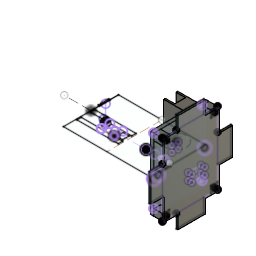
Slider Gear and Screw Box (Autodesk Fusion 360 design; units mm, degrees)
description: Spur Gear; Module: 3.0; Num Teeth: 12; Pressure Angle: 20.0; Backlash: 0.00 mm
part number: 2026-03-27-17-39-36-868
Autodesk Fusion 360 part; units mm, degrees
(part 1 of 2)
sketch "Base Circle" plane through (0, 0, 0) normal (0, 0, 1) x (1, 0, 0)
  circle A0 centre (0, 0) radius 14.529
  circle A1 centre (0, 0) radius 1.75
  dimension "d22" = 3.5
  measures "d22" diameter of A1
extrude "Extrude1" add sketch "Base Circle" along normal blind 8 makes body 1
sketch "Gear Tooth" plane through (0, 0, 0) normal (0, 0, 1) x (1, 0, 0)
  spline S0 degree 5 poles (16.735, -2.4575) (16.7471, -2.4592) (16.7712, -2.4624) (16.8075, -2.466) (16.8561, -2.4685) (16.9171, -2.4687) (16.9782, -2.4667) (17.0395, -2.4633) (17.1009, -2.4593) (17.1623, -2.4548) (17.2237, -2.4497) (17.2852, -2.4439) (17.3467, -2.4372) (17.4083, -2.4294) (17.4699, -2.4206) (17.5316, -2.4107) (17.5933, -2.4) (17.6549, -2.3886) (17.7166, -2.3766) (17.7783, -2.364) (17.84, -2.3508) (17.9017, -2.337) (17.9634, -2.3225) (18.025, -2.3073) (18.0867, -2.2914) (18.1483, -2.2749) (18.2099, -2.2578) (18.2715, -2.2401) (18.3331, -2.2219) (18.3946, -2.2031) (18.4561, -2.1837) (18.5175, -2.1638) (18.579, -2.1433) (18.6403, -2.1223) (18.7017, -2.1007) (18.763, -2.0786) (18.8242, -2.056) (18.8854, -2.0329) (18.9465, -2.0092) (19.0076, -1.9851) (19.0686, -1.9605) (19.1296, -1.9353) (19.1905, -1.9097) (19.2514, -1.8836) (19.3121, -1.857) (19.3728, -1.8299) (19.4335, -1.8024) (19.494, -1.7743) (19.5545, -1.7459) (19.615, -1.7169) (19.6753, -1.6875) (19.7355, -1.6577) (19.7957, -1.6274) (19.8558, -1.5966) (19.9158, -1.5654) (19.9757, -1.5338) (20.0356, -1.5017) (20.0953, -1.4692) (20.155, -1.4362) (20.2145, -1.4029) (20.274, -1.3691) (20.3333, -1.3348) (20.3926, -1.3002) (20.4518, -1.2651) (20.5108, -1.2296) (20.5698, -1.1937) (20.6286, -1.1574) (20.6874, -1.1207) (20.746, -1.0836) (20.8045, -1.0461) (20.8629, -1.0082) (20.9095, -0.9775) (20.9445, -0.9544) (20.9677, -0.9388) (20.9794, -0.931) knots 0 0 0 0 0 0 0.01428571 0.02857143 0.04285714 0.05714286 0.07142857 0.08571429 0.1 0.11428571 0.12857143 0.14285714 0.15714286 0.17142857 0.18571429 0.2 0.21428571 0.22857143 0.24285714 0.25714286 0.27142857 0.28571429 0.3 0.31428571 0.32857143 0.34285714 0.35714286 0.37142857 0.38571429 0.4 0.41428571 0.42857143 0.44285714 0.45714286 0.47142857 0.48571429 0.5 0.51428571 0.52857143 0.54285714 0.55714286 0.57142857 0.58571429 0.6 0.61428571 0.62857143 0.64285714 0.65714286 0.67142857 0.68571429 0.7 0.71428571 0.72857143 0.74285714 0.75714286 0.77142857 0.78571429 0.8 0.81428571 0.82857143 0.84285714 0.85714286 0.87142857 0.88571429 0.9 0.91428571 0.92857143 0.94285714 0.95714286 0.97142857 0.98571429 1 1 1 1 1 1
  spline S1 degree 5 poles (16.735, 2.4575) (16.7471, 2.4592) (16.7712, 2.4624) (16.8075, 2.466) (16.8561, 2.4685) (16.9171, 2.4687) (16.9782, 2.4667) (17.0395, 2.4633) (17.1009, 2.4593) (17.1623, 2.4548) (17.2237, 2.4497) (17.2852, 2.4439) (17.3467, 2.4372) (17.4083, 2.4294) (17.4699, 2.4206) (17.5316, 2.4107) (17.5933, 2.4) (17.6549, 2.3886) (17.7166, 2.3766) (17.7783, 2.364) (17.84, 2.3508) (17.9017, 2.337) (17.9634, 2.3225) (18.025, 2.3073) (18.0867, 2.2914) (18.1483, 2.2749) (18.2099, 2.2578) (18.2715, 2.2401) (18.3331, 2.2219) (18.3946, 2.2031) (18.4561, 2.1837) (18.5175, 2.1638) (18.579, 2.1433) (18.6403, 2.1223) (18.7017, 2.1007) (18.763, 2.0786) (18.8242, 2.056) (18.8854, 2.0329) (18.9465, 2.0092) (19.0076, 1.9851) (19.0686, 1.9605) (19.1296, 1.9353) (19.1905, 1.9097) (19.2514, 1.8836) (19.3121, 1.857) (19.3728, 1.8299) (19.4335, 1.8024) (19.494, 1.7743) (19.5545, 1.7459) (19.615, 1.7169) (19.6753, 1.6875) (19.7355, 1.6577) (19.7957, 1.6274) (19.8558, 1.5966) (19.9158, 1.5654) (19.9757, 1.5338) (20.0356, 1.5017) (20.0953, 1.4692) (20.155, 1.4362) (20.2145, 1.4029) (20.274, 1.3691) (20.3333, 1.3348) (20.3926, 1.3002) (20.4518, 1.2651) (20.5108, 1.2296) (20.5698, 1.1937) (20.6286, 1.1574) (20.6874, 1.1207) (20.746, 1.0836) (20.8045, 1.0461) (20.8629, 1.0082) (20.9095, 0.9775) (20.9445, 0.9544) (20.9677, 0.9388) (20.9794, 0.931) knots 0 0 0 0 0 0 0.01428571 0.02857143 0.04285714 0.05714286 0.07142857 0.08571429 0.1 0.11428571 0.12857143 0.14285714 0.15714286 0.17142857 0.18571429 0.2 0.21428571 0.22857143 0.24285714 0.25714286 0.27142857 0.28571429 0.3 0.31428571 0.32857143 0.34285714 0.35714286 0.37142857 0.38571429 0.4 0.41428571 0.42857143 0.44285714 0.45714286 0.47142857 0.48571429 0.5 0.51428571 0.52857143 0.54285714 0.55714286 0.57142857 0.58571429 0.6 0.61428571 0.62857143 0.64285714 0.65714286 0.67142857 0.68571429 0.7 0.71428571 0.72857143 0.74285714 0.75714286 0.77142857 0.78571429 0.8 0.81428571 0.82857143 0.84285714 0.85714286 0.87142857 0.88571429 0.9 0.91428571 0.92857143 0.94285714 0.95714286 0.97142857 0.98571429 1 1 1 1 1 1
  arc A0 (20.9794, -0.931) -> (20.9794, 0.931) centre (0, 0) ccw
  line L0 (14.3649, -2.1094) -> (16.735, -2.4575)
  line L1 (14.3649, 2.1094) -> (16.735, 2.4575)
  line L2 (14.3649, -2.1094) -> (14.3649, 2.1094)
  point P0 (17.029, -2.4638)
  point P1 (17.3273, -2.4392)
  point P2 (17.6282, -2.3935)
  point P3 (17.931, -2.33)
  point P4 (18.2352, -2.2505)
  point P5 (18.5405, -2.1561)
  point P6 (18.8463, -2.0476)
  point P7 (19.1525, -1.9256)
  point P8 (19.4587, -1.7906)
  point P9 (19.7645, -1.643)
  point P10 (20.0698, -1.483)
  point P11 (20.3742, -1.3109)
  point P12 (20.6775, -1.1268)
  point P13 (17.029, 2.4638)
  point P14 (17.3273, 2.4392)
  point P15 (17.6282, 2.3935)
  point P16 (17.931, 2.33)
  point P17 (18.2352, 2.2505)
  point P18 (18.5405, 2.1561)
  point P19 (18.8463, 2.0476)
  point P20 (19.1525, 1.9256)
  point P21 (19.4587, 1.7906)
  point P22 (19.7645, 1.643)
  point P23 (20.0698, 1.483)
  point P24 (20.3742, 1.3109)
  point P25 (20.6775, 1.1268)
extrude "Extrude2" add sketch "Gear Tooth" along normal blind 8 bodies 1
fillet "Fillet1" radius 1 2 edges at (14.3748, -2.1109, 4) (14.3748, 2.1109, 4) on bodies 1
pattern_circular "C-Pattern1" count 12 over 360 about axis through (0, 0, 0) along (0, 0, 1) of "Extrude2", "Fillet1"
sketch "Diametrial Pitch Circle" plane through (0, 0, 0) normal (0, 0, 1) x (1, 0, 0)
  circle A0 centre (0, 0) radius 18 construction
sketch "Connecting Rod" plane through (0, 0, 8) normal (0, 0, 1) x (-1, 0, 0)
  arc A0 (-13.8215, 4.4786) -> (-14.2091, 3.0322) centre (0, 0) ccw
  arc A1 (-15.3323, 2.2515) -> (-14.2091, 3.0322) centre (-15.1871, 3.2409) ccw
  line L0 (-15.3323, 2.2515) -> (-16.735, 2.4575)
  spline S0 degree 5 poles (-16.735, 2.4575) (-16.7471, 2.4592) (-16.7712, 2.4624) (-16.8075, 2.466) (-16.8561, 2.4685) (-16.9171, 2.4687) (-16.9782, 2.4667) (-17.0395, 2.4633) (-17.1009, 2.4593) (-17.1623, 2.4548) (-17.2237, 2.4497) (-17.2852, 2.4439) (-17.3467, 2.4372) (-17.4083, 2.4294) (-17.4699, 2.4206) (-17.5316, 2.4107) (-17.5933, 2.4) (-17.6549, 2.3886) (-17.7166, 2.3766) (-17.7783, 2.364) (-17.84, 2.3508) (-17.9017, 2.337) (-17.9634, 2.3225) (-18.025, 2.3073) (-18.0867, 2.2914) (-18.1483, 2.2749) (-18.2099, 2.2578) (-18.2715, 2.2401) (-18.3331, 2.2219) (-18.3946, 2.2031) (-18.4561, 2.1837) (-18.5175, 2.1638) (-18.579, 2.1433) (-18.6403, 2.1223) (-18.7017, 2.1007) (-18.763, 2.0786) (-18.8242, 2.056) (-18.8854, 2.0329) (-18.9465, 2.0092) (-19.0076, 1.9851) (-19.0686, 1.9605) (-19.1296, 1.9353) (-19.1905, 1.9097) (-19.2514, 1.8836) (-19.3121, 1.857) (-19.3728, 1.8299) (-19.4335, 1.8024) (-19.494, 1.7743) (-19.5545, 1.7459) (-19.615, 1.7169) (-19.6753, 1.6875) (-19.7355, 1.6577) (-19.7957, 1.6274) (-19.8558, 1.5966) (-19.9158, 1.5654) (-19.9757, 1.5338) (-20.0356, 1.5017) (-20.0953, 1.4692) (-20.155, 1.4362) (-20.2145, 1.4029) (-20.274, 1.3691) (-20.3333, 1.3348) (-20.3926, 1.3002) (-20.4518, 1.2651) (-20.5108, 1.2296) (-20.5698, 1.1937) (-20.6286, 1.1574) (-20.6874, 1.1207) (-20.746, 1.0836) (-20.8045, 1.0461) (-20.8629, 1.0082) (-20.9095, 0.9775) (-20.9445, 0.9544) (-20.9677, 0.9388) (-20.9794, 0.931) knots 0 0 0 0 0 0 0.01428571 0.02857143 0.04285714 0.05714286 0.07142857 0.08571429 0.1 0.11428571 0.12857143 0.14285714 0.15714286 0.17142857 0.18571429 0.2 0.21428571 0.22857143 0.24285714 0.25714286 0.27142857 0.28571429 0.3 0.31428571 0.32857143 0.34285714 0.35714286 0.37142857 0.38571429 0.4 0.41428571 0.42857143 0.44285714 0.45714286 0.47142857 0.48571429 0.5 0.51428571 0.52857143 0.54285714 0.55714286 0.57142857 0.58571429 0.6 0.61428571 0.62857143 0.64285714 0.65714286 0.67142857 0.68571429 0.7 0.71428571 0.72857143 0.74285714 0.75714286 0.77142857 0.78571429 0.8 0.81428571 0.82857143 0.84285714 0.85714286 0.87142857 0.88571429 0.9 0.91428571 0.92857143 0.94285714 0.95714286 0.97142857 0.98571429 1 1 1 1 1 1
  arc A2 (-20.9794, 0.931) -> (-20.9794, -0.931) centre (0, 0) ccw
  spline S1 degree 5 poles (-20.9794, -0.931) (-20.9677, -0.9388) (-20.9445, -0.9544) (-20.9095, -0.9775) (-20.8629, -1.0082) (-20.8045, -1.0461) (-20.746, -1.0836) (-20.6874, -1.1207) (-20.6286, -1.1574) (-20.5698, -1.1937) (-20.5108, -1.2296) (-20.4518, -1.2651) (-20.3926, -1.3002) (-20.3333, -1.3348) (-20.274, -1.3691) (-20.2145, -1.4029) (-20.155, -1.4362) (-20.0953, -1.4692) (-20.0356, -1.5017) (-19.9757, -1.5338) (-19.9158, -1.5654) (-19.8558, -1.5966) (-19.7957, -1.6274) (-19.7355, -1.6577) (-19.6753, -1.6875) (-19.615, -1.7169) (-19.5545, -1.7459) (-19.494, -1.7743) (-19.4335, -1.8024) (-19.3728, -1.8299) (-19.3121, -1.857) (-19.2514, -1.8836) (-19.1905, -1.9097) (-19.1296, -1.9353) (-19.0686, -1.9605) (-19.0076, -1.9851) (-18.9465, -2.0092) (-18.8854, -2.0329) (-18.8242, -2.056) (-18.763, -2.0786) (-18.7017, -2.1007) (-18.6403, -2.1223) (-18.579, -2.1433) (-18.5175, -2.1638) (-18.4561, -2.1837) (-18.3946, -2.2031) (-18.3331, -2.2219) (-18.2715, -2.2401) (-18.2099, -2.2578) (-18.1483, -2.2749) (-18.0867, -2.2914) (-18.025, -2.3073) (-17.9634, -2.3225) (-17.9017, -2.337) (-17.84, -2.3508) (-17.7783, -2.364) (-17.7166, -2.3766) (-17.6549, -2.3886) (-17.5933, -2.4) (-17.5316, -2.4107) (-17.4699, -2.4206) (-17.4083, -2.4294) (-17.3467, -2.4372) (-17.2852, -2.4439) (-17.2237, -2.4497) (-17.1623, -2.4548) (-17.1009, -2.4593) (-17.0395, -2.4633) (-16.9782, -2.4667) (-16.9171, -2.4687) (-16.8561, -2.4685) (-16.8075, -2.466) (-16.7712, -2.4624) (-16.7471, -2.4592) (-16.735, -2.4575) knots -1 -1 -1 -1 -1 -1 -0.98571429 -0.97142857 -0.95714286 -0.94285714 -0.92857143 -0.91428571 -0.9 -0.88571429 -0.87142857 -0.85714286 -0.84285714 -0.82857143 -0.81428571 -0.8 -0.78571429 -0.77142857 -0.75714286 -0.74285714 -0.72857143 -0.71428571 -0.7 -0.68571429 -0.67142857 -0.65714286 -0.64285714 -0.62857143 -0.61428571 -0.6 -0.58571429 -0.57142857 -0.55714286 -0.54285714 -0.52857143 -0.51428571 -0.5 -0.48571429 -0.47142857 -0.45714286 -0.44285714 -0.42857143 -0.41428571 -0.4 -0.38571429 -0.37142857 -0.35714286 -0.34285714 -0.32857143 -0.31428571 -0.3 -0.28571429 -0.27142857 -0.25714286 -0.24285714 -0.22857143 -0.21428571 -0.2 -0.18571429 -0.17142857 -0.15714286 -0.14285714 -0.12857143 -0.11428571 -0.1 -0.08571429 -0.07142857 -0.05714286 -0.04285714 -0.02857143 -0.01428571 0 0 0 0 0 0
  line L1 (-16.735, -2.4575) -> (-15.3323, -2.2515)
  arc A3 (-14.2091, -3.0322) -> (-15.3323, -2.2515) centre (-15.1871, -3.2409) ccw
  arc A4 (-14.4039, -5.7163) -> (-13.8215, -4.4786) centre (-14.7728, -4.7868) ccw
  line L2 (-14.4039, -5.7163) -> (-15.7217, -6.2393)
  spline S2 degree 5 poles (-15.7217, -6.2393) (-15.733, -6.2438) (-15.7555, -6.2531) (-15.7887, -6.2682) (-15.8321, -6.2903) (-15.885, -6.3206) (-15.9369, -6.3529) (-15.9883, -6.3864) (-16.0394, -6.4206) (-16.0903, -6.4553) (-16.141, -6.4904) (-16.1914, -6.5261) (-16.2413, -6.5627) (-16.2907, -6.6002) (-16.3397, -6.6387) (-16.3882, -6.678) (-16.4362, -6.7181) (-16.4839, -6.7588) (-16.5314, -6.8001) (-16.5785, -6.8418) (-16.6253, -6.8841) (-16.6718, -6.927) (-16.718, -6.9703) (-16.7638, -7.0143) (-16.8092, -7.0589) (-16.8544, -7.104) (-16.8992, -7.1496) (-16.9436, -7.1957) (-16.9878, -7.2423) (-17.0317, -7.2894) (-17.0753, -7.3369) (-17.1185, -7.3849) (-17.1615, -7.4333) (-17.2042, -7.4822) (-17.2465, -7.5315) (-17.2885, -7.5813) (-17.3303, -7.6315) (-17.3717, -7.6822) (-17.4128, -7.7332) (-17.4536, -7.7847) (-17.4942, -7.8365) (-17.5344, -7.8888) (-17.5743, -7.9414) (-17.614, -7.9944) (-17.6533, -8.0479) (-17.6923, -8.1017) (-17.7311, -8.1559) (-17.7695, -8.2104) (-17.8077, -8.2653) (-17.8455, -8.3206) (-17.8831, -8.3762) (-17.9203, -8.4322) (-17.9573, -8.4885) (-17.9939, -8.5452) (-18.0303, -8.6022) (-18.0664, -8.6596) (-18.1022, -8.7173) (-18.1376, -8.7753) (-18.1728, -8.8337) (-18.2077, -8.8924) (-18.2423, -8.9514) (-18.2766, -9.0107) (-18.3106, -9.0703) (-18.3443, -9.1303) (-18.3777, -9.1905) (-18.4108, -9.2511) (-18.4436, -9.3119) (-18.4761, -9.3731) (-18.5084, -9.4345) (-18.5403, -9.4963) (-18.5719, -9.5583) (-18.597, -9.6082) (-18.6156, -9.6457) (-18.628, -9.6708) (-18.6342, -9.6834) knots 0 0 0 0 0 0 0.01428571 0.02857143 0.04285714 0.05714286 0.07142857 0.08571429 0.1 0.11428571 0.12857143 0.14285714 0.15714286 0.17142857 0.18571429 0.2 0.21428571 0.22857143 0.24285714 0.25714286 0.27142857 0.28571429 0.3 0.31428571 0.32857143 0.34285714 0.35714286 0.37142857 0.38571429 0.4 0.41428571 0.42857143 0.44285714 0.45714286 0.47142857 0.48571429 0.5 0.51428571 0.52857143 0.54285714 0.55714286 0.57142857 0.58571429 0.6 0.61428571 0.62857143 0.64285714 0.65714286 0.67142857 0.68571429 0.7 0.71428571 0.72857143 0.74285714 0.75714286 0.77142857 0.78571429 0.8 0.81428571 0.82857143 0.84285714 0.85714286 0.87142857 0.88571429 0.9 0.91428571 0.92857143 0.94285714 0.95714286 0.97142857 0.98571429 1 1 1 1 1 1
  arc A5 (-18.6342, -9.6834) -> (-17.7031, -11.296) centre (0, 0) ccw
  spline S3 degree 5 poles (-17.7031, -11.296) (-17.6892, -11.2969) (-17.6613, -11.2987) (-17.6194, -11.3013) (-17.5637, -11.3046) (-17.4942, -11.3082) (-17.4247, -11.3114) (-17.3554, -11.3143) (-17.2862, -11.3167) (-17.2171, -11.3187) (-17.1481, -11.3203) (-17.0792, -11.3215) (-17.0104, -11.3223) (-16.9418, -11.3227) (-16.8733, -11.3226) (-16.8049, -11.3222) (-16.7366, -11.3213) (-16.6685, -11.32) (-16.6005, -11.3183) (-16.5326, -11.3161) (-16.4649, -11.3136) (-16.3973, -11.3106) (-16.3299, -11.3072) (-16.2627, -11.3033) (-16.1955, -11.2991) (-16.1286, -11.2944) (-16.0618, -11.2892) (-15.9952, -11.2836) (-15.9287, -11.2776) (-15.8624, -11.2712) (-15.7963, -11.2643) (-15.7304, -11.2569) (-15.6646, -11.2491) (-15.5991, -11.2408) (-15.5337, -11.2321) (-15.4685, -11.223) (-15.4036, -11.2133) (-15.3388, -11.2032) (-15.2742, -11.1927) (-15.2099, -11.1816) (-15.1458, -11.1701) (-15.0819, -11.1581) (-15.0182, -11.1456) (-14.9548, -11.1327) (-14.8916, -11.1192) (-14.8286, -11.1052) (-14.766, -11.0907) (-14.7035, -11.0758) (-14.6413, -11.0603) (-14.5794, -11.0443) (-14.5178, -11.0278) (-14.4565, -11.0107) (-14.3955, -10.993) (-14.3348, -10.9747) (-14.2745, -10.9559) (-14.2145, -10.9365) (-14.1547, -10.9165) (-14.0953, -10.8961) (-14.0362, -10.8751) (-13.9774, -10.8535) (-13.9191, -10.8312) (-13.8613, -10.8081) (-13.8041, -10.7841) (-13.7475, -10.7591) (-13.6913, -10.7334) (-13.6356, -10.707) (-13.5801, -10.6803) (-13.525, -10.6531) (-13.4703, -10.6253) (-13.4163, -10.5965) (-13.3636, -10.5658) (-13.3228, -10.5393) (-13.2931, -10.5181) (-13.2738, -10.5033) (-13.2642, -10.4957) knots -1 -1 -1 -1 -1 -1 -0.98571429 -0.97142857 -0.95714286 -0.94285714 -0.92857143 -0.91428571 -0.9 -0.88571429 -0.87142857 -0.85714286 -0.84285714 -0.82857143 -0.81428571 -0.8 -0.78571429 -0.77142857 -0.75714286 -0.74285714 -0.72857143 -0.71428571 -0.7 -0.68571429 -0.67142857 -0.65714286 -0.64285714 -0.62857143 -0.61428571 -0.6 -0.58571429 -0.57142857 -0.55714286 -0.54285714 -0.52857143 -0.51428571 -0.5 -0.48571429 -0.47142857 -0.45714286 -0.44285714 -0.42857143 -0.41428571 -0.4 -0.38571429 -0.37142857 -0.35714286 -0.34285714 -0.32857143 -0.31428571 -0.3 -0.28571429 -0.27142857 -0.25714286 -0.24285714 -0.22857143 -0.21428571 -0.2 -0.18571429 -0.17142857 -0.15714286 -0.14285714 -0.12857143 -0.11428571 -0.1 -0.08571429 -0.07142857 -0.05714286 -0.04285714 -0.02857143 -0.01428571 0 0 0 0 0 0
  line L3 (-13.2642, -10.4957) -> (-12.1524, -9.616)
  arc A6 (-10.7893, -9.7305) -> (-12.1524, -9.616) centre (-11.5319, -10.4002) ccw
  arc A7 (-9.616, -12.1524) -> (-9.7305, -10.7893) centre (-10.4002, -11.5319) ccw
  line L4 (-9.616, -12.1524) -> (-10.4957, -13.2642)
  spline S4 degree 5 poles (-10.4957, -13.2642) (-10.5033, -13.2738) (-10.5181, -13.2931) (-10.5393, -13.3228) (-10.5658, -13.3636) (-10.5965, -13.4163) (-10.6253, -13.4703) (-10.6531, -13.525) (-10.6803, -13.5801) (-10.707, -13.6356) (-10.7334, -13.6913) (-10.7591, -13.7475) (-10.7841, -13.8041) (-10.8081, -13.8613) (-10.8312, -13.9191) (-10.8535, -13.9774) (-10.8751, -14.0362) (-10.8961, -14.0953) (-10.9165, -14.1547) (-10.9365, -14.2145) (-10.9559, -14.2745) (-10.9747, -14.3348) (-10.993, -14.3955) (-11.0107, -14.4565) (-11.0278, -14.5178) (-11.0443, -14.5794) (-11.0603, -14.6413) (-11.0758, -14.7035) (-11.0907, -14.766) (-11.1052, -14.8286) (-11.1192, -14.8916) (-11.1327, -14.9548) (-11.1456, -15.0182) (-11.1581, -15.0819) (-11.1701, -15.1458) (-11.1816, -15.2099) (-11.1927, -15.2742) (-11.2032, -15.3388) (-11.2133, -15.4036) (-11.223, -15.4685) (-11.2321, -15.5337) (-11.2408, -15.5991) (-11.2491, -15.6646) (-11.2569, -15.7304) (-11.2643, -15.7963) (-11.2712, -15.8624) (-11.2776, -15.9287) (-11.2836, -15.9952) (-11.2892, -16.0618) (-11.2944, -16.1286) (-11.2991, -16.1955) (-11.3033, -16.2627) (-11.3072, -16.3299) (-11.3106, -16.3973) (-11.3136, -16.4649) (-11.3161, -16.5326) (-11.3183, -16.6005) (-11.32, -16.6685) (-11.3213, -16.7366) (-11.3222, -16.8049) (-11.3226, -16.8733) (-11.3227, -16.9418) (-11.3223, -17.0104) (-11.3215, -17.0792) (-11.3203, -17.1481) (-11.3187, -17.2171) (-11.3167, -17.2862) (-11.3143, -17.3554) (-11.3114, -17.4247) (-11.3082, -17.4942) (-11.3046, -17.5637) (-11.3013, -17.6194) (-11.2987, -17.6613) (-11.2969, -17.6892) (-11.296, -17.7031) knots 0 0 0 0 0 0 0.01428571 0.02857143 0.04285714 0.05714286 0.07142857 0.08571429 0.1 0.11428571 0.12857143 0.14285714 0.15714286 0.17142857 0.18571429 0.2 0.21428571 0.22857143 0.24285714 0.25714286 0.27142857 0.28571429 0.3 0.31428571 0.32857143 0.34285714 0.35714286 0.37142857 0.38571429 0.4 0.41428571 0.42857143 0.44285714 0.45714286 0.47142857 0.48571429 0.5 0.51428571 0.52857143 0.54285714 0.55714286 0.57142857 0.58571429 0.6 0.61428571 0.62857143 0.64285714 0.65714286 0.67142857 0.68571429 0.7 0.71428571 0.72857143 0.74285714 0.75714286 0.77142857 0.78571429 0.8 0.81428571 0.82857143 0.84285714 0.85714286 0.87142857 0.88571429 0.9 0.91428571 0.92857143 0.94285714 0.95714286 0.97142857 0.98571429 1 1 1 1 1 1
  arc A8 (-11.296, -17.7031) -> (-9.6834, -18.6342) centre (0, 0) ccw
  spline S5 degree 5 poles (-9.6834, -18.6342) (-9.6708, -18.628) (-9.6457, -18.6156) (-9.6082, -18.597) (-9.5583, -18.5719) (-9.4963, -18.5403) (-9.4345, -18.5084) (-9.3731, -18.4761) (-9.3119, -18.4436) (-9.2511, -18.4108) (-9.1905, -18.3777) (-9.1303, -18.3443) (-9.0703, -18.3106) (-9.0107, -18.2766) (-8.9514, -18.2423) (-8.8924, -18.2077) (-8.8337, -18.1728) (-8.7753, -18.1376) (-8.7173, -18.1022) (-8.6596, -18.0664) (-8.6022, -18.0303) (-8.5452, -17.9939) (-8.4885, -17.9573) (-8.4322, -17.9203) (-8.3762, -17.8831) (-8.3206, -17.8455) (-8.2653, -17.8077) (-8.2104, -17.7695) (-8.1559, -17.7311) (-8.1017, -17.6923) (-8.0479, -17.6533) (-7.9944, -17.614) (-7.9414, -17.5743) (-7.8888, -17.5344) (-7.8365, -17.4942) (-7.7847, -17.4536) (-7.7332, -17.4128) (-7.6822, -17.3717) (-7.6315, -17.3303) (-7.5813, -17.2885) (-7.5315, -17.2465) (-7.4822, -17.2042) (-7.4333, -17.1615) (-7.3849, -17.1185) (-7.3369, -17.0753) (-7.2894, -17.0317) (-7.2423, -16.9878) (-7.1957, -16.9436) (-7.1496, -16.8992) (-7.104, -16.8544) (-7.0589, -16.8092) (-7.0143, -16.7638) (-6.9703, -16.718) (-6.927, -16.6718) (-6.8841, -16.6253) (-6.8418, -16.5785) (-6.8001, -16.5314) (-6.7588, -16.4839) (-6.7181, -16.4362) (-6.678, -16.3882) (-6.6387, -16.3397) (-6.6002, -16.2907) (-6.5627, -16.2413) (-6.5261, -16.1914) (-6.4904, -16.141) (-6.4553, -16.0903) (-6.4206, -16.0394) (-6.3864, -15.9883) (-6.3529, -15.9369) (-6.3206, -15.885) (-6.2903, -15.8321) (-6.2682, -15.7887) (-6.2531, -15.7555) (-6.2438, -15.733) (-6.2393, -15.7217) knots -1 -1 -1 -1 -1 -1 -0.98571429 -0.97142857 -0.95714286 -0.94285714 -0.92857143 -0.91428571 -0.9 -0.88571429 -0.87142857 -0.85714286 -0.84285714 -0.82857143 -0.81428571 -0.8 -0.78571429 -0.77142857 -0.75714286 -0.74285714 -0.72857143 -0.71428571 -0.7 -0.68571429 -0.67142857 -0.65714286 -0.64285714 -0.62857143 -0.61428571 -0.6 -0.58571429 -0.57142857 -0.55714286 -0.54285714 -0.52857143 -0.51428571 -0.5 -0.48571429 -0.47142857 -0.45714286 -0.44285714 -0.42857143 -0.41428571 -0.4 -0.38571429 -0.37142857 -0.35714286 -0.34285714 -0.32857143 -0.31428571 -0.3 -0.28571429 -0.27142857 -0.25714286 -0.24285714 -0.22857143 -0.21428571 -0.2 -0.18571429 -0.17142857 -0.15714286 -0.14285714 -0.12857143 -0.11428571 -0.1 -0.08571429 -0.07142857 -0.05714286 -0.04285714 -0.02857143 -0.01428571 0 0 0 0 0 0
  line L5 (-6.2393, -15.7217) -> (-5.7163, -14.4039)
  arc A9 (-4.4786, -13.8215) -> (-5.7163, -14.4039) centre (-4.7868, -14.7728) ccw
  arc A10 (-2.2515, -15.3323) -> (-3.0322, -14.2091) centre (-3.2409, -15.1871) ccw
  line L6 (-2.2515, -15.3323) -> (-2.4575, -16.735)
  spline S6 degree 5 poles (-2.4575, -16.735) (-2.4592, -16.7471) (-2.4624, -16.7712) (-2.466, -16.8075) (-2.4685, -16.8561) (-2.4687, -16.9171) (-2.4667, -16.9782) (-2.4633, -17.0395) (-2.4593, -17.1009) (-2.4548, -17.1623) (-2.4497, -17.2237) (-2.4439, -17.2852) (-2.4372, -17.3467) (-2.4294, -17.4083) (-2.4206, -17.4699) (-2.4107, -17.5316) (-2.4, -17.5933) (-2.3886, -17.6549) (-2.3766, -17.7166) (-2.364, -17.7783) (-2.3508, -17.84) (-2.337, -17.9017) (-2.3225, -17.9634) (-2.3073, -18.025) (-2.2914, -18.0867) (-2.2749, -18.1483) (-2.2578, -18.2099) (-2.2401, -18.2715) (-2.2219, -18.3331) (-2.2031, -18.3946) (-2.1837, -18.4561) (-2.1638, -18.5175) (-2.1433, -18.579) (-2.1223, -18.6403) (-2.1007, -18.7017) (-2.0786, -18.763) (-2.056, -18.8242) (-2.0329, -18.8854) (-2.0092, -18.9465) (-1.9851, -19.0076) (-1.9605, -19.0686) (-1.9353, -19.1296) (-1.9097, -19.1905) (-1.8836, -19.2514) (-1.857, -19.3121) (-1.8299, -19.3728) (-1.8024, -19.4335) (-1.7743, -19.494) (-1.7459, -19.5545) (-1.7169, -19.615) (-1.6875, -19.6753) (-1.6577, -19.7355) (-1.6274, -19.7957) (-1.5966, -19.8558) (-1.5654, -19.9158) (-1.5338, -19.9757) (-1.5017, -20.0356) (-1.4692, -20.0953) (-1.4362, -20.155) (-1.4029, -20.2145) (-1.3691, -20.274) (-1.3348, -20.3333) (-1.3002, -20.3926) (-1.2651, -20.4518) (-1.2296, -20.5108) (-1.1937, -20.5698) (-1.1574, -20.6286) (-1.1207, -20.6874) (-1.0836, -20.746) (-1.0461, -20.8045) (-1.0082, -20.8629) (-0.9775, -20.9095) (-0.9544, -20.9445) (-0.9388, -20.9677) (-0.931, -20.9794) knots 0 0 0 0 0 0 0.01428571 0.02857143 0.04285714 0.05714286 0.07142857 0.08571429 0.1 0.11428571 0.12857143 0.14285714 0.15714286 0.17142857 0.18571429 0.2 0.21428571 0.22857143 0.24285714 0.25714286 0.27142857 0.28571429 0.3 0.31428571 0.32857143 0.34285714 0.35714286 0.37142857 0.38571429 0.4 0.41428571 0.42857143 0.44285714 0.45714286 0.47142857 0.48571429 0.5 0.51428571 0.52857143 0.54285714 0.55714286 0.57142857 0.58571429 0.6 0.61428571 0.62857143 0.64285714 0.65714286 0.67142857 0.68571429 0.7 0.71428571 0.72857143 0.74285714 0.75714286 0.77142857 0.78571429 0.8 0.81428571 0.82857143 0.84285714 0.85714286 0.87142857 0.88571429 0.9 0.91428571 0.92857143 0.94285714 0.95714286 0.97142857 0.98571429 1 1 1 1 1 1
  arc A11 (-0.931, -20.9794) -> (0.931, -20.9794) centre (0, 0) ccw
  spline S7 degree 5 poles (0.931, -20.9794) (0.9388, -20.9677) (0.9544, -20.9445) (0.9775, -20.9095) (1.0082, -20.8629) (1.0461, -20.8045) (1.0836, -20.746) (1.1207, -20.6874) (1.1574, -20.6286) (1.1937, -20.5698) (1.2296, -20.5108) (1.2651, -20.4518) (1.3002, -20.3926) (1.3348, -20.3333) (1.3691, -20.274) (1.4029, -20.2145) (1.4362, -20.155) (1.4692, -20.0953) (1.5017, -20.0356) (1.5338, -19.9757) (1.5654, -19.9158) (1.5966, -19.8558) (1.6274, -19.7957) (1.6577, -19.7355) (1.6875, -19.6753) (1.7169, -19.615) (1.7459, -19.5545) (1.7743, -19.494) (1.8024, -19.4335) (1.8299, -19.3728) (1.857, -19.3121) (1.8836, -19.2514) (1.9097, -19.1905) (1.9353, -19.1296) (1.9605, -19.0686) (1.9851, -19.0076) (2.0092, -18.9465) (2.0329, -18.8854) (2.056, -18.8242) (2.0786, -18.763) (2.1007, -18.7017) (2.1223, -18.6403) (2.1433, -18.579) (2.1638, -18.5175) (2.1837, -18.4561) (2.2031, -18.3946) (2.2219, -18.3331) (2.2401, -18.2715) (2.2578, -18.2099) (2.2749, -18.1483) (2.2914, -18.0867) (2.3073, -18.025) (2.3225, -17.9634) (2.337, -17.9017) (2.3508, -17.84) (2.364, -17.7783) (2.3766, -17.7166) (2.3886, -17.6549) (2.4, -17.5933) (2.4107, -17.5316) (2.4206, -17.4699) (2.4294, -17.4083) (2.4372, -17.3467) (2.4439, -17.2852) (2.4497, -17.2237) (2.4548, -17.1623) (2.4593, -17.1009) (2.4633, -17.0395) (2.4667, -16.9782) (2.4687, -16.9171) (2.4685, -16.8561) (2.466, -16.8075) (2.4624, -16.7712) (2.4592, -16.7471) (2.4575, -16.735) knots -1 -1 -1 -1 -1 -1 -0.98571429 -0.97142857 -0.95714286 -0.94285714 -0.92857143 -0.91428571 -0.9 -0.88571429 -0.87142857 -0.85714286 -0.84285714 -0.82857143 -0.81428571 -0.8 -0.78571429 -0.77142857 -0.75714286 -0.74285714 -0.72857143 -0.71428571 -0.7 -0.68571429 -0.67142857 -0.65714286 -0.64285714 -0.62857143 -0.61428571 -0.6 -0.58571429 -0.57142857 -0.55714286 -0.54285714 -0.52857143 -0.51428571 -0.5 -0.48571429 -0.47142857 -0.45714286 -0.44285714 -0.42857143 -0.41428571 -0.4 -0.38571429 -0.37142857 -0.35714286 -0.34285714 -0.32857143 -0.31428571 -0.3 -0.28571429 -0.27142857 -0.25714286 -0.24285714 -0.22857143 -0.21428571 -0.2 -0.18571429 -0.17142857 -0.15714286 -0.14285714 -0.12857143 -0.11428571 -0.1 -0.08571429 -0.07142857 -0.05714286 -0.04285714 -0.02857143 -0.01428571 0 0 0 0 0 0
  line L7 (2.4575, -16.735) -> (2.2515, -15.3323)
  arc A12 (3.0322, -14.2091) -> (2.2515, -15.3323) centre (3.2409, -15.1871) ccw
  arc A13 (5.7163, -14.4039) -> (4.4786, -13.8215) centre (4.7868, -14.7728) ccw
  line L8 (5.7163, -14.4039) -> (6.2393, -15.7217)
  spline S8 degree 5 poles (6.2393, -15.7217) (6.2438, -15.733) (6.2531, -15.7555) (6.2682, -15.7887) (6.2903, -15.8321) (6.3206, -15.885) (6.3529, -15.9369) (6.3864, -15.9883) (6.4206, -16.0394) (6.4553, -16.0903) (6.4904, -16.141) (6.5261, -16.1914) (6.5627, -16.2413) (6.6002, -16.2907) (6.6387, -16.3397) (6.678, -16.3882) (6.7181, -16.4362) (6.7588, -16.4839) (6.8001, -16.5314) (6.8418, -16.5785) (6.8841, -16.6253) (6.927, -16.6718) (6.9703, -16.718) (7.0143, -16.7638) (7.0589, -16.8092) (7.104, -16.8544) (7.1496, -16.8992) (7.1957, -16.9436) (7.2423, -16.9878) (7.2894, -17.0317) (7.3369, -17.0753) (7.3849, -17.1185) (7.4333, -17.1615) (7.4822, -17.2042) (7.5315, -17.2465) (7.5813, -17.2885) (7.6315, -17.3303) (7.6822, -17.3717) (7.7332, -17.4128) (7.7847, -17.4536) (7.8365, -17.4942) (7.8888, -17.5344) (7.9414, -17.5743) (7.9944, -17.614) (8.0479, -17.6533) (8.1017, -17.6923) (8.1559, -17.7311) (8.2104, -17.7695) (8.2653, -17.8077) (8.3206, -17.8455) (8.3762, -17.8831) (8.4322, -17.9203) (8.4885, -17.9573) (8.5452, -17.9939) (8.6022, -18.0303) (8.6596, -18.0664) (8.7173, -18.1022) (8.7753, -18.1376) (8.8337, -18.1728) (8.8924, -18.2077) (8.9514, -18.2423) (9.0107, -18.2766) (9.0703, -18.3106) (9.1303, -18.3443) (9.1905, -18.3777) (9.2511, -18.4108) (9.3119, -18.4436) (9.3731, -18.4761) (9.4345, -18.5084) (9.4963, -18.5403) (9.5583, -18.5719) (9.6082, -18.597) (9.6457, -18.6156) (9.6708, -18.628) (9.6834, -18.6342) knots 0 0 0 0 0 0 0.01428571 0.02857143 0.04285714 0.05714286 0.07142857 0.08571429 0.1 0.11428571 0.12857143 0.14285714 0.15714286 0.17142857 0.18571429 0.2 0.21428571 0.22857143 0.24285714 0.25714286 0.27142857 0.28571429 0.3 0.31428571 0.32857143 0.34285714 0.35714286 0.37142857 0.38571429 0.4 0.41428571 0.42857143 0.44285714 0.45714286 0.47142857 0.48571429 0.5 0.51428571 0.52857143 0.54285714 0.55714286 0.57142857 0.58571429 0.6 0.61428571 0.62857143 0.64285714 0.65714286 0.67142857 0.68571429 0.7 0.71428571 0.72857143 0.74285714 0.75714286 0.77142857 0.78571429 0.8 0.81428571 0.82857143 0.84285714 0.85714286 0.87142857 0.88571429 0.9 0.91428571 0.92857143 0.94285714 0.95714286 0.97142857 0.98571429 1 1 1 1 1 1
  arc A14 (9.6834, -18.6342) -> (11.296, -17.7031) centre (0, 0) ccw
  spline S9 degree 5 poles (11.296, -17.7031) (11.2969, -17.6892) (11.2987, -17.6613) (11.3013, -17.6194) (11.3046, -17.5637) (11.3082, -17.4942) (11.3114, -17.4247) (11.3143, -17.3554) (11.3167, -17.2862) (11.3187, -17.2171) (11.3203, -17.1481) (11.3215, -17.0792) (11.3223, -17.0104) (11.3227, -16.9418) (11.3226, -16.8733) (11.3222, -16.8049) (11.3213, -16.7366) (11.32, -16.6685) (11.3183, -16.6005) (11.3161, -16.5326) (11.3136, -16.4649) (11.3106, -16.3973) (11.3072, -16.3299) (11.3033, -16.2627) (11.2991, -16.1955) (11.2944, -16.1286) (11.2892, -16.0618) (11.2836, -15.9952) (11.2776, -15.9287) (11.2712, -15.8624) (11.2643, -15.7963) (11.2569, -15.7304) (11.2491, -15.6646) (11.2408, -15.5991) (11.2321, -15.5337) (11.223, -15.4685) (11.2133, -15.4036) (11.2032, -15.3388) (11.1927, -15.2742) (11.1816, -15.2099) (11.1701, -15.1458) (11.1581, -15.0819) (11.1456, -15.0182) (11.1327, -14.9548) (11.1192, -14.8916) (11.1052, -14.8286) (11.0907, -14.766) (11.0758, -14.7035) (11.0603, -14.6413) (11.0443, -14.5794) (11.0278, -14.5178) (11.0107, -14.4565) (10.993, -14.3955) (10.9747, -14.3348) (10.9559, -14.2745) (10.9365, -14.2145) (10.9165, -14.1547) (10.8961, -14.0953) (10.8751, -14.0362) (10.8535, -13.9774) (10.8312, -13.9191) (10.8081, -13.8613) (10.7841, -13.8041) (10.7591, -13.7475) (10.7334, -13.6913) (10.707, -13.6356) (10.6803, -13.5801) (10.6531, -13.525) (10.6253, -13.4703) (10.5965, -13.4163) (10.5658, -13.3636) (10.5393, -13.3228) (10.5181, -13.2931) (10.5033, -13.2738) (10.4957, -13.2642) knots -1 -1 -1 -1 -1 -1 -0.98571429 -0.97142857 -0.95714286 -0.94285714 -0.92857143 -0.91428571 -0.9 -0.88571429 -0.87142857 -0.85714286 -0.84285714 -0.82857143 -0.81428571 -0.8 -0.78571429 -0.77142857 -0.75714286 -0.74285714 -0.72857143 -0.71428571 -0.7 -0.68571429 -0.67142857 -0.65714286 -0.64285714 -0.62857143 -0.61428571 -0.6 -0.58571429 -0.57142857 -0.55714286 -0.54285714 -0.52857143 -0.51428571 -0.5 -0.48571429 -0.47142857 -0.45714286 -0.44285714 -0.42857143 -0.41428571 -0.4 -0.38571429 -0.37142857 -0.35714286 -0.34285714 -0.32857143 -0.31428571 -0.3 -0.28571429 -0.27142857 -0.25714286 -0.24285714 -0.22857143 -0.21428571 -0.2 -0.18571429 -0.17142857 -0.15714286 -0.14285714 -0.12857143 -0.11428571 -0.1 -0.08571429 -0.07142857 -0.05714286 -0.04285714 -0.02857143 -0.01428571 0 0 0 0 0 0
  line L9 (10.4957, -13.2642) -> (9.616, -12.1524)
  arc A15 (9.7305, -10.7893) -> (9.616, -12.1524) centre (10.4002, -11.5319) ccw
  arc A16 (12.1524, -9.616) -> (10.7893, -9.7305) centre (11.5319, -10.4002) ccw
  line L10 (12.1524, -9.616) -> (13.2642, -10.4957)
  spline S10 degree 5 poles (13.2642, -10.4957) (13.2738, -10.5033) (13.2931, -10.5181) (13.3228, -10.5393) (13.3636, -10.5658) (13.4163, -10.5965) (13.4703, -10.6253) (13.525, -10.6531) (13.5801, -10.6803) (13.6356, -10.707) (13.6913, -10.7334) (13.7475, -10.7591) (13.8041, -10.7841) (13.8613, -10.8081) (13.9191, -10.8312) (13.9774, -10.8535) (14.0362, -10.8751) (14.0953, -10.8961) (14.1547, -10.9165) (14.2145, -10.9365) (14.2745, -10.9559) (14.3348, -10.9747) (14.3955, -10.993) (14.4565, -11.0107) (14.5178, -11.0278) (14.5794, -11.0443) (14.6413, -11.0603) (14.7035, -11.0758) (14.766, -11.0907) (14.8286, -11.1052) (14.8916, -11.1192) (14.9548, -11.1327) (15.0182, -11.1456) (15.0819, -11.1581) (15.1458, -11.1701) (15.2099, -11.1816) (15.2742, -11.1927) (15.3388, -11.2032) (15.4036, -11.2133) (15.4685, -11.223) (15.5337, -11.2321) (15.5991, -11.2408) (15.6646, -11.2491) (15.7304, -11.2569) (15.7963, -11.2643) (15.8624, -11.2712) (15.9287, -11.2776) (15.9952, -11.2836) (16.0618, -11.2892) (16.1286, -11.2944) (16.1955, -11.2991) (16.2627, -11.3033) (16.3299, -11.3072) (16.3973, -11.3106) (16.4649, -11.3136) (16.5326, -11.3161) (16.6005, -11.3183) (16.6685, -11.32) (16.7366, -11.3213) (16.8049, -11.3222) (16.8733, -11.3226) (16.9418, -11.3227) (17.0104, -11.3223) (17.0792, -11.3215) (17.1481, -11.3203) (17.2171, -11.3187) (17.2862, -11.3167) (17.3554, -11.3143) (17.4247, -11.3114) (17.4942, -11.3082) (17.5637, -11.3046) (17.6194, -11.3013) (17.6613, -11.2987) (17.6892, -11.2969) (17.7031, -11.296) knots 0 0 0 0 0 0 0.01428571 0.02857143 0.04285714 0.05714286 0.07142857 0.08571429 0.1 0.11428571 0.12857143 0.14285714 0.15714286 0.17142857 0.18571429 0.2 0.21428571 0.22857143 0.24285714 0.25714286 0.27142857 0.28571429 0.3 0.31428571 0.32857143 0.34285714 0.35714286 0.37142857 0.38571429 0.4 0.41428571 0.42857143 0.44285714 0.45714286 0.47142857 0.48571429 0.5 0.51428571 0.52857143 0.54285714 0.55714286 0.57142857 0.58571429 0.6 0.61428571 0.62857143 0.64285714 0.65714286 0.67142857 0.68571429 0.7 0.71428571 0.72857143 0.74285714 0.75714286 0.77142857 0.78571429 0.8 0.81428571 0.82857143 0.84285714 0.85714286 0.87142857 0.88571429 0.9 0.91428571 0.92857143 0.94285714 0.95714286 0.97142857 0.98571429 1 1 1 1 1 1
  arc A17 (17.7031, -11.296) -> (18.6342, -9.6834) centre (0, 0) ccw
  spline S11 degree 5 poles (18.6342, -9.6834) (18.628, -9.6708) (18.6156, -9.6457) (18.597, -9.6082) (18.5719, -9.5583) (18.5403, -9.4963) (18.5084, -9.4345) (18.4761, -9.3731) (18.4436, -9.3119) (18.4108, -9.2511) (18.3777, -9.1905) (18.3443, -9.1303) (18.3106, -9.0703) (18.2766, -9.0107) (18.2423, -8.9514) (18.2077, -8.8924) (18.1728, -8.8337) (18.1376, -8.7753) (18.1022, -8.7173) (18.0664, -8.6596) (18.0303, -8.6022) (17.9939, -8.5452) (17.9573, -8.4885) (17.9203, -8.4322) (17.8831, -8.3762) (17.8455, -8.3206) (17.8077, -8.2653) (17.7695, -8.2104) (17.7311, -8.1559) (17.6923, -8.1017) (17.6533, -8.0479) (17.614, -7.9944) (17.5743, -7.9414) (17.5344, -7.8888) (17.4942, -7.8365) (17.4536, -7.7847) (17.4128, -7.7332) (17.3717, -7.6822) (17.3303, -7.6315) (17.2885, -7.5813) (17.2465, -7.5315) (17.2042, -7.4822) (17.1615, -7.4333) (17.1185, -7.3849) (17.0753, -7.3369) (17.0317, -7.2894) (16.9878, -7.2423) (16.9436, -7.1957) (16.8992, -7.1496) (16.8544, -7.104) (16.8092, -7.0589) (16.7638, -7.0143) (16.718, -6.9703) (16.6718, -6.927) (16.6253, -6.8841) (16.5785, -6.8418) (16.5314, -6.8001) (16.4839, -6.7588) (16.4362, -6.7181) (16.3882, -6.678) (16.3397, -6.6387) (16.2907, -6.6002) (16.2413, -6.5627) (16.1914, -6.5261) (16.141, -6.4904) (16.0903, -6.4553) (16.0394, -6.4206) (15.9883, -6.3864) (15.9369, -6.3529) (15.885, -6.3206) (15.8321, -6.2903) (15.7887, -6.2682) (15.7555, -6.2531) (15.733, -6.2438) (15.7217, -6.2393) knots -1 -1 -1 -1 -1 -1 -0.98571429 -0.97142857 -0.95714286 -0.94285714 -0.92857143 -0.91428571 -0.9 -0.88571429 -0.87142857 -0.85714286 -0.84285714 -0.82857143 -0.81428571 -0.8 -0.78571429 -0.77142857 -0.75714286 -0.74285714 -0.72857143 -0.71428571 -0.7 -0.68571429 -0.67142857 -0.65714286 -0.64285714 -0.62857143 -0.61428571 -0.6 -0.58571429 -0.57142857 -0.55714286 -0.54285714 -0.52857143 -0.51428571 -0.5 -0.48571429 -0.47142857 -0.45714286 -0.44285714 -0.42857143 -0.41428571 -0.4 -0.38571429 -0.37142857 -0.35714286 -0.34285714 -0.32857143 -0.31428571 -0.3 -0.28571429 -0.27142857 -0.25714286 -0.24285714 -0.22857143 -0.21428571 -0.2 -0.18571429 -0.17142857 -0.15714286 -0.14285714 -0.12857143 -0.11428571 -0.1 -0.08571429 -0.07142857 -0.05714286 -0.04285714 -0.02857143 -0.01428571 0 0 0 0 0 0
  line L11 (15.7217, -6.2393) -> (14.4039, -5.7163)
  arc A18 (13.8215, -4.4786) -> (14.4039, -5.7163) centre (14.7728, -4.7868) ccw
  arc A19 (15.3323, -2.2515) -> (14.2091, -3.0322) centre (15.1871, -3.2409) ccw
  line L12 (15.3323, -2.2515) -> (16.735, -2.4575)
  spline S12 degree 5 poles (16.735, -2.4575) (16.7471, -2.4592) (16.7712, -2.4624) (16.8075, -2.466) (16.8561, -2.4685) (16.9171, -2.4687) (16.9782, -2.4667) (17.0395, -2.4633) (17.1009, -2.4593) (17.1623, -2.4548) (17.2237, -2.4497) (17.2852, -2.4439) (17.3467, -2.4372) (17.4083, -2.4294) (17.4699, -2.4206) (17.5316, -2.4107) (17.5933, -2.4) (17.6549, -2.3886) (17.7166, -2.3766) (17.7783, -2.364) (17.84, -2.3508) (17.9017, -2.337) (17.9634, -2.3225) (18.025, -2.3073) (18.0867, -2.2914) (18.1483, -2.2749) (18.2099, -2.2578) (18.2715, -2.2401) (18.3331, -2.2219) (18.3946, -2.2031) (18.4561, -2.1837) (18.5175, -2.1638) (18.579, -2.1433) (18.6403, -2.1223) (18.7017, -2.1007) (18.763, -2.0786) (18.8242, -2.056) (18.8854, -2.0329) (18.9465, -2.0092) (19.0076, -1.9851) (19.0686, -1.9605) (19.1296, -1.9353) (19.1905, -1.9097) (19.2514, -1.8836) (19.3121, -1.857) (19.3728, -1.8299) (19.4335, -1.8024) (19.494, -1.7743) (19.5545, -1.7459) (19.615, -1.7169) (19.6753, -1.6875) (19.7355, -1.6577) (19.7957, -1.6274) (19.8558, -1.5966) (19.9158, -1.5654) (19.9757, -1.5338) (20.0356, -1.5017) (20.0953, -1.4692) (20.155, -1.4362) (20.2145, -1.4029) (20.274, -1.3691) (20.3333, -1.3348) (20.3926, -1.3002) (20.4518, -1.2651) (20.5108, -1.2296) (20.5698, -1.1937) (20.6286, -1.1574) (20.6874, -1.1207) (20.746, -1.0836) (20.8045, -1.0461) (20.8629, -1.0082) (20.9095, -0.9775) (20.9445, -0.9544) (20.9677, -0.9388) (20.9794, -0.931) knots 0 0 0 0 0 0 0.01428571 0.02857143 0.04285714 0.05714286 0.07142857 0.08571429 0.1 0.11428571 0.12857143 0.14285714 0.15714286 0.17142857 0.18571429 0.2 0.21428571 0.22857143 0.24285714 0.25714286 0.27142857 0.28571429 0.3 0.31428571 0.32857143 0.34285714 0.35714286 0.37142857 0.38571429 0.4 0.41428571 0.42857143 0.44285714 0.45714286 0.47142857 0.48571429 0.5 0.51428571 0.52857143 0.54285714 0.55714286 0.57142857 0.58571429 0.6 0.61428571 0.62857143 0.64285714 0.65714286 0.67142857 0.68571429 0.7 0.71428571 0.72857143 0.74285714 0.75714286 0.77142857 0.78571429 0.8 0.81428571 0.82857143 0.84285714 0.85714286 0.87142857 0.88571429 0.9 0.91428571 0.92857143 0.94285714 0.95714286 0.97142857 0.98571429 1 1 1 1 1 1
  arc A20 (20.9794, -0.931) -> (20.9794, 0.931) centre (0, 0) ccw
  spline S13 degree 5 poles (20.9794, 0.931) (20.9677, 0.9388) (20.9445, 0.9544) (20.9095, 0.9775) (20.8629, 1.0082) (20.8045, 1.0461) (20.746, 1.0836) (20.6874, 1.1207) (20.6286, 1.1574) (20.5698, 1.1937) (20.5108, 1.2296) (20.4518, 1.2651) (20.3926, 1.3002) (20.3333, 1.3348) (20.274, 1.3691) (20.2145, 1.4029) (20.155, 1.4362) (20.0953, 1.4692) (20.0356, 1.5017) (19.9757, 1.5338) (19.9158, 1.5654) (19.8558, 1.5966) (19.7957, 1.6274) (19.7355, 1.6577) (19.6753, 1.6875) (19.615, 1.7169) (19.5545, 1.7459) (19.494, 1.7743) (19.4335, 1.8024) (19.3728, 1.8299) (19.3121, 1.857) (19.2514, 1.8836) (19.1905, 1.9097) (19.1296, 1.9353) (19.0686, 1.9605) (19.0076, 1.9851) (18.9465, 2.0092) (18.8854, 2.0329) (18.8242, 2.056) (18.763, 2.0786) (18.7017, 2.1007) (18.6403, 2.1223) (18.579, 2.1433) (18.5175, 2.1638) (18.4561, 2.1837) (18.3946, 2.2031) (18.3331, 2.2219) (18.2715, 2.2401) (18.2099, 2.2578) (18.1483, 2.2749) (18.0867, 2.2914) (18.025, 2.3073) (17.9634, 2.3225) (17.9017, 2.337) (17.84, 2.3508) (17.7783, 2.364) (17.7166, 2.3766) (17.6549, 2.3886) (17.5933, 2.4) (17.5316, 2.4107) (17.4699, 2.4206) (17.4083, 2.4294) (17.3467, 2.4372) (17.2852, 2.4439) (17.2237, 2.4497) (17.1623, 2.4548) (17.1009, 2.4593) (17.0395, 2.4633) (16.9782, 2.4667) (16.9171, 2.4687) (16.8561, 2.4685) (16.8075, 2.466) (16.7712, 2.4624) (16.7471, 2.4592) (16.735, 2.4575) knots -1 -1 -1 -1 -1 -1 -0.98571429 -0.97142857 -0.95714286 -0.94285714 -0.92857143 -0.91428571 -0.9 -0.88571429 -0.87142857 -0.85714286 -0.84285714 -0.82857143 -0.81428571 -0.8 -0.78571429 -0.77142857 -0.75714286 -0.74285714 -0.72857143 -0.71428571 -0.7 -0.68571429 -0.67142857 -0.65714286 -0.64285714 -0.62857143 -0.61428571 -0.6 -0.58571429 -0.57142857 -0.55714286 -0.54285714 -0.52857143 -0.51428571 -0.5 -0.48571429 -0.47142857 -0.45714286 -0.44285714 -0.42857143 -0.41428571 -0.4 -0.38571429 -0.37142857 -0.35714286 -0.34285714 -0.32857143 -0.31428571 -0.3 -0.28571429 -0.27142857 -0.25714286 -0.24285714 -0.22857143 -0.21428571 -0.2 -0.18571429 -0.17142857 -0.15714286 -0.14285714 -0.12857143 -0.11428571 -0.1 -0.08571429 -0.07142857 -0.05714286 -0.04285714 -0.02857143 -0.01428571 0 0 0 0 0 0
  line L13 (16.735, 2.4575) -> (15.3323, 2.2515)
  arc A21 (14.2091, 3.0322) -> (15.3323, 2.2515) centre (15.1871, 3.2409) ccw
  arc A22 (14.4039, 5.7163) -> (13.8215, 4.4786) centre (14.7728, 4.7868) ccw
  line L14 (14.4039, 5.7163) -> (15.7217, 6.2393)
  spline S14 degree 5 poles (15.7217, 6.2393) (15.733, 6.2438) (15.7555, 6.2531) (15.7887, 6.2682) (15.8321, 6.2903) (15.885, 6.3206) (15.9369, 6.3529) (15.9883, 6.3864) (16.0394, 6.4206) (16.0903, 6.4553) (16.141, 6.4904) (16.1914, 6.5261) (16.2413, 6.5627) (16.2907, 6.6002) (16.3397, 6.6387) (16.3882, 6.678) (16.4362, 6.7181) (16.4839, 6.7588) (16.5314, 6.8001) (16.5785, 6.8418) (16.6253, 6.8841) (16.6718, 6.927) (16.718, 6.9703) (16.7638, 7.0143) (16.8092, 7.0589) (16.8544, 7.104) (16.8992, 7.1496) (16.9436, 7.1957) (16.9878, 7.2423) (17.0317, 7.2894) (17.0753, 7.3369) (17.1185, 7.3849) (17.1615, 7.4333) (17.2042, 7.4822) (17.2465, 7.5315) (17.2885, 7.5813) (17.3303, 7.6315) (17.3717, 7.6822) (17.4128, 7.7332) (17.4536, 7.7847) (17.4942, 7.8365) (17.5344, 7.8888) (17.5743, 7.9414) (17.614, 7.9944) (17.6533, 8.0479) (17.6923, 8.1017) (17.7311, 8.1559) (17.7695, 8.2104) (17.8077, 8.2653) (17.8455, 8.3206) (17.8831, 8.3762) (17.9203, 8.4322) (17.9573, 8.4885) (17.9939, 8.5452) (18.0303, 8.6022) (18.0664, 8.6596) (18.1022, 8.7173) (18.1376, 8.7753) (18.1728, 8.8337) (18.2077, 8.8924) (18.2423, 8.9514) (18.2766, 9.0107) (18.3106, 9.0703) (18.3443, 9.1303) (18.3777, 9.1905) (18.4108, 9.2511) (18.4436, 9.3119) (18.4761, 9.3731) (18.5084, 9.4345) (18.5403, 9.4963) (18.5719, 9.5583) (18.597, 9.6082) (18.6156, 9.6457) (18.628, 9.6708) (18.6342, 9.6834) knots 0 0 0 0 0 0 0.01428571 0.02857143 0.04285714 0.05714286 0.07142857 0.08571429 0.1 0.11428571 0.12857143 0.14285714 0.15714286 0.17142857 0.18571429 0.2 0.21428571 0.22857143 0.24285714 0.25714286 0.27142857 0.28571429 0.3 0.31428571 0.32857143 0.34285714 0.35714286 0.37142857 0.38571429 0.4 0.41428571 0.42857143 0.44285714 0.45714286 0.47142857 0.48571429 0.5 0.51428571 0.52857143 0.54285714 0.55714286 0.57142857 0.58571429 0.6 0.61428571 0.62857143 0.64285714 0.65714286 0.67142857 0.68571429 0.7 0.71428571 0.72857143 0.74285714 0.75714286 0.77142857 0.78571429 0.8 0.81428571 0.82857143 0.84285714 0.85714286 0.87142857 0.88571429 0.9 0.91428571 0.92857143 0.94285714 0.95714286 0.97142857 0.98571429 1 1 1 1 1 1
  arc A23 (18.6342, 9.6834) -> (17.7031, 11.296) centre (0, 0) ccw
  spline S15 degree 5 poles (17.7031, 11.296) (17.6892, 11.2969) (17.6613, 11.2987) (17.6194, 11.3013) (17.5637, 11.3046) (17.4942, 11.3082) (17.4247, 11.3114) (17.3554, 11.3143) (17.2862, 11.3167) (17.2171, 11.3187) (17.1481, 11.3203) (17.0792, 11.3215) (17.0104, 11.3223) (16.9418, 11.3227) (16.8733, 11.3226) (16.8049, 11.3222) (16.7366, 11.3213) (16.6685, 11.32) (16.6005, 11.3183) (16.5326, 11.3161) (16.4649, 11.3136) (16.3973, 11.3106) (16.3299, 11.3072) (16.2627, 11.3033) (16.1955, 11.2991) (16.1286, 11.2944) (16.0618, 11.2892) (15.9952, 11.2836) (15.9287, 11.2776) (15.8624, 11.2712) (15.7963, 11.2643) (15.7304, 11.2569) (15.6646, 11.2491) (15.5991, 11.2408) (15.5337, 11.2321) (15.4685, 11.223) (15.4036, 11.2133) (15.3388, 11.2032) (15.2742, 11.1927) (15.2099, 11.1816) (15.1458, 11.1701) (15.0819, 11.1581) (15.0182, 11.1456) (14.9548, 11.1327) (14.8916, 11.1192) (14.8286, 11.1052) (14.766, 11.0907) (14.7035, 11.0758) (14.6413, 11.0603) (14.5794, 11.0443) (14.5178, 11.0278) (14.4565, 11.0107) (14.3955, 10.993) (14.3348, 10.9747) (14.2745, 10.9559) (14.2145, 10.9365) (14.1547, 10.9165) (14.0953, 10.8961) (14.0362, 10.8751) (13.9774, 10.8535) (13.9191, 10.8312) (13.8613, 10.8081) (13.8041, 10.7841) (13.7475, 10.7591) (13.6913, 10.7334) (13.6356, 10.707) (13.5801, 10.6803) (13.525, 10.6531) (13.4703, 10.6253) (13.4163, 10.5965) (13.3636, 10.5658) (13.3228, 10.5393) (13.2931, 10.5181) (13.2738, 10.5033) (13.2642, 10.4957) knots -1 -1 -1 -1 -1 -1 -0.98571429 -0.97142857 -0.95714286 -0.94285714 -0.92857143 -0.91428571 -0.9 -0.88571429 -0.87142857 -0.85714286 -0.84285714 -0.82857143 -0.81428571 -0.8 -0.78571429 -0.77142857 -0.75714286 -0.74285714 -0.72857143 -0.71428571 -0.7 -0.68571429 -0.67142857 -0.65714286 -0.64285714 -0.62857143 -0.61428571 -0.6 -0.58571429 -0.57142857 -0.55714286 -0.54285714 -0.52857143 -0.51428571 -0.5 -0.48571429 -0.47142857 -0.45714286 -0.44285714 -0.42857143 -0.41428571 -0.4 -0.38571429 -0.37142857 -0.35714286 -0.34285714 -0.32857143 -0.31428571 -0.3 -0.28571429 -0.27142857 -0.25714286 -0.24285714 -0.22857143 -0.21428571 -0.2 -0.18571429 -0.17142857 -0.15714286 -0.14285714 -0.12857143 -0.11428571 -0.1 -0.08571429 -0.07142857 -0.05714286 -0.04285714 -0.02857143 -0.01428571 0 0 0 0 0 0
  line L15 (13.2642, 10.4957) -> (12.1524, 9.616)
  arc A24 (10.7893, 9.7305) -> (12.1524, 9.616) centre (11.5319, 10.4002) ccw
  arc A25 (9.616, 12.1524) -> (9.7305, 10.7893) centre (10.4002, 11.5319) ccw
  line L16 (9.616, 12.1524) -> (10.4957, 13.2642)
  spline S16 degree 5 poles (10.4957, 13.2642) (10.5033, 13.2738) (10.5181, 13.2931) (10.5393, 13.3228) (10.5658, 13.3636) (10.5965, 13.4163) (10.6253, 13.4703) (10.6531, 13.525) (10.6803, 13.5801) (10.707, 13.6356) (10.7334, 13.6913) (10.7591, 13.7475) (10.7841, 13.8041) (10.8081, 13.8613) (10.8312, 13.9191) (10.8535, 13.9774) (10.8751, 14.0362) (10.8961, 14.0953) (10.9165, 14.1547) (10.9365, 14.2145) (10.9559, 14.2745) (10.9747, 14.3348) (10.993, 14.3955) (11.0107, 14.4565) (11.0278, 14.5178) (11.0443, 14.5794) (11.0603, 14.6413) (11.0758, 14.7035) (11.0907, 14.766) (11.1052, 14.8286) (11.1192, 14.8916) (11.1327, 14.9548) (11.1456, 15.0182) (11.1581, 15.0819) (11.1701, 15.1458) (11.1816, 15.2099) (11.1927, 15.2742) (11.2032, 15.3388) (11.2133, 15.4036) (11.223, 15.4685) (11.2321, 15.5337) (11.2408, 15.5991) (11.2491, 15.6646) (11.2569, 15.7304) (11.2643, 15.7963) (11.2712, 15.8624) (11.2776, 15.9287) (11.2836, 15.9952) (11.2892, 16.0618) (11.2944, 16.1286) (11.2991, 16.1955) (11.3033, 16.2627) (11.3072, 16.3299) (11.3106, 16.3973) (11.3136, 16.4649) (11.3161, 16.5326) (11.3183, 16.6005) (11.32, 16.6685) (11.3213, 16.7366) (11.3222, 16.8049) (11.3226, 16.8733) (11.3227, 16.9418) (11.3223, 17.0104) (11.3215, 17.0792) (11.3203, 17.1481) (11.3187, 17.2171) (11.3167, 17.2862) (11.3143, 17.3554) (11.3114, 17.4247) (11.3082, 17.4942) (11.3046, 17.5637) (11.3013, 17.6194) (11.2987, 17.6613) (11.2969, 17.6892) (11.296, 17.7031) knots 0 0 0 0 0 0 0.01428571 0.02857143 0.04285714 0.05714286 0.07142857 0.08571429 0.1 0.11428571 0.12857143 0.14285714 0.15714286 0.17142857 0.18571429 0.2 0.21428571 0.22857143 0.24285714 0.25714286 0.27142857 0.28571429 0.3 0.31428571 0.32857143 0.34285714 0.35714286 0.37142857 0.38571429 0.4 0.41428571 0.42857143 0.44285714 0.45714286 0.47142857 0.48571429 0.5 0.51428571 0.52857143 0.54285714 0.55714286 0.57142857 0.58571429 0.6 0.61428571 0.62857143 0.64285714 0.65714286 0.67142857 0.68571429 0.7 0.71428571 0.72857143 0.74285714 0.75714286 0.77142857 0.78571429 0.8 0.81428571 0.82857143 0.84285714 0.85714286 0.87142857 0.88571429 0.9 0.91428571 0.92857143 0.94285714 0.95714286 0.97142857 0.98571429 1 1 1 1 1 1
  arc A26 (11.296, 17.7031) -> (9.6834, 18.6342) centre (0, 0) ccw
  spline S17 degree 5 poles (9.6834, 18.6342) (9.6708, 18.628) (9.6457, 18.6156) (9.6082, 18.597) (9.5583, 18.5719) (9.4963, 18.5403) (9.4345, 18.5084) (9.3731, 18.4761) (9.3119, 18.4436) (9.2511, 18.4108) (9.1905, 18.3777) (9.1303, 18.3443) (9.0703, 18.3106) (9.0107, 18.2766) (8.9514, 18.2423) (8.8924, 18.2077) (8.8337, 18.1728) (8.7753, 18.1376) (8.7173, 18.1022) (8.6596, 18.0664) (8.6022, 18.0303) (8.5452, 17.9939) (8.4885, 17.9573) (8.4322, 17.9203) (8.3762, 17.8831) (8.3206, 17.8455) (8.2653, 17.8077) (8.2104, 17.7695) (8.1559, 17.7311) (8.1017, 17.6923) (8.0479, 17.6533) (7.9944, 17.614) (7.9414, 17.5743) (7.8888, 17.5344) (7.8365, 17.4942) (7.7847, 17.4536) (7.7332, 17.4128) (7.6822, 17.3717) (7.6315, 17.3303) (7.5813, 17.2885) (7.5315, 17.2465) (7.4822, 17.2042) (7.4333, 17.1615) (7.3849, 17.1185) (7.3369, 17.0753) (7.2894, 17.0317) (7.2423, 16.9878) (7.1957, 16.9436) (7.1496, 16.8992) (7.104, 16.8544) (7.0589, 16.8092) (7.0143, 16.7638) (6.9703, 16.718) (6.927, 16.6718) (6.8841, 16.6253) (6.8418, 16.5785) (6.8001, 16.5314) (6.7588, 16.4839) (6.7181, 16.4362) (6.678, 16.3882) (6.6387, 16.3397) (6.6002, 16.2907) (6.5627, 16.2413) (6.5261, 16.1914) (6.4904, 16.141) (6.4553, 16.0903) (6.4206, 16.0394) (6.3864, 15.9883) (6.3529, 15.9369) (6.3206, 15.885) (6.2903, 15.8321) (6.2682, 15.7887) (6.2531, 15.7555) (6.2438, 15.733) (6.2393, 15.7217) knots -1 -1 -1 -1 -1 -1 -0.98571429 -0.97142857 -0.95714286 -0.94285714 -0.92857143 -0.91428571 -0.9 -0.88571429 -0.87142857 -0.85714286 -0.84285714 -0.82857143 -0.81428571 -0.8 -0.78571429 -0.77142857 -0.75714286 -0.74285714 -0.72857143 -0.71428571 -0.7 -0.68571429 -0.67142857 -0.65714286 -0.64285714 -0.62857143 -0.61428571 -0.6 -0.58571429 -0.57142857 -0.55714286 -0.54285714 -0.52857143 -0.51428571 -0.5 -0.48571429 -0.47142857 -0.45714286 -0.44285714 -0.42857143 -0.41428571 -0.4 -0.38571429 -0.37142857 -0.35714286 -0.34285714 -0.32857143 -0.31428571 -0.3 -0.28571429 -0.27142857 -0.25714286 -0.24285714 -0.22857143 -0.21428571 -0.2 -0.18571429 -0.17142857 -0.15714286 -0.14285714 -0.12857143 -0.11428571 -0.1 -0.08571429 -0.07142857 -0.05714286 -0.04285714 -0.02857143 -0.01428571 0 0 0 0 0 0
  line L17 (6.2393, 15.7217) -> (5.7163, 14.4039)
  arc A27 (4.4786, 13.8215) -> (5.7163, 14.4039) centre (4.7868, 14.7728) ccw
  arc A28 (2.2515, 15.3323) -> (3.0322, 14.2091) centre (3.2409, 15.1871) ccw
  line L18 (2.2515, 15.3323) -> (2.4575, 16.735)